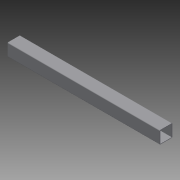
# Autodesk Inventor part: 24_inch_square
Saved by Autodesk Inventor 2015 SP1 (Build 190203100, 203)
## iProperties
Created: 2016-02-03
Part Number: 24_inch_square
Material: Generic
Document SubType Name: Modeling
Designer: guillemd
Density: 1 g/cm^3
Appearance: Default
Author: guillemd
Autodesk Inventor part; units mm, degrees
ref_plane "YZ Plane" through (0, 0, 0) normal (1, 0, 0) x (0, 1, 0)
ref_plane "XZ Plane" through (0, 0, 0) normal (0, 1, 0) x (-1, 0, 0)
ref_plane "XY Plane" through (0, 0, 0) normal (0, 0, 1) x (1, 0, 0)
sketch "Sketch1" plane through (0, 0, 0) normal (1, 0, 0) x (0, 1, 0)
  line L0 (25.4, 25.4) -> (-25.4, 25.4)
  line L1 (-25.4, 25.4) -> (-25.4, -25.4)
  line L2 (-25.4, -25.4) -> (25.4, -25.4)
  line L3 (25.4, -25.4) -> (25.4, 25.4)
  line L4 (23.2918, 23.2918) -> (-23.2918, 23.2918)
  line L5 (-23.2918, 23.2918) -> (-23.2918, -23.2918)
  line L6 (-23.2918, -23.2918) -> (23.2918, -23.2918)
  line L7 (23.2918, -23.2918) -> (23.2918, 23.2918)
  point P0 (0, 0)
  point P1 (0, -25.4)
  point P2 (25.4, 0)
  dimension "d0" = 50.8
  dimension "d1" = 50.8
  dimension "d2" = 2.1082
  constraints: 16 end point, 4 parallel, 2 midpoint, 2 perpendicular, 1 horizontal, 1 horizontal alignment, 1 vertical alignment, 3 other
  measures "d0" distance of L1.end L2.end
  measures "d1" distance of L2.end L0.start
  measures "d2" distance between parallel lines of L3 L7
extrude "Extrusion1" add sketch "Sketch1" along normal blind 609.6
fillet "Fillet1" radius 3.175 4 edges at (304.8, 25.4, 25.4) (304.8, -25.4, 25.4) (304.8, 25.4, -25.4) (304.8, -25.4, -25.4)
body "Solid1"
